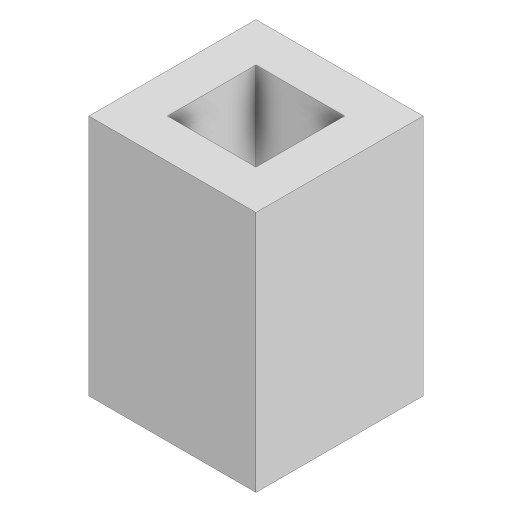
# Autodesk Inventor part: Tampa_fotometro
Saved by Autodesk Inventor 2024.3 (Build 283343000, 343)
## iProperties
Created: 2024-05-16
Part Number: Tampa_fotometro
Material: Genérico
Document SubType Name: Modeling
Designer: barof
Density: 1 g/cm^3
Appearance: Padrão
Author: barof
## iProperties of the stored document Tampa_fotometro_3DPrint.ipt
Created: 2025-02-10
Part Number: Tampa_fotometro_3DPrint
Material: Genérico
Document SubType Name: Modeling
Designer: barof
Density: 1 g/cm^3
Appearance: Padrão
Author: barof
Autodesk Inventor part; units mm, degrees
ref_plane "YZ Plane" through (0, 0, 0) normal (1, 0, 0) x (0, 1, 0)
ref_plane "XZ Plane" through (0, 0, 0) normal (0, 1, 0) x (-1, 0, 0)
ref_plane "XY Plane" through (0, 0, 0) normal (0, 0, 1) x (1, 0, 0)
sketch "Esboço1" plane through (0, 0, 0) normal (0, 1, 0) x (-1, 0, 0)
  line L0 (0, 0) -> (-25.5, 0)
  line L1 (-25.5, 0) -> (-25.5, -25.5)
  line L2 (-25.5, -25.5) -> (0, -25.5)
  line L3 (0, -25.5) -> (0, 0)
  line L4 (-6, -19.5) -> (-19.5, -19.5)
  line L5 (-19.5, -19.5) -> (-19.5, -6)
  line L6 (-19.5, -6) -> (-6, -6)
  line L7 (-6, -6) -> (-6, -19.5)
  point P0 (-25.5, -12.75)
  point P1 (-19.5, -12.75)
  point P2 (-12.75, 0)
  point P3 (-12.75, -6)
  point P4 (-6, -12.75)
  dimension "d0" = 6
  dimension "d1" = 6
  dimension "d2" = 6
  dimension "d3" = 6
  dimension "d4" = 13.5
  dimension "d5" = 13.5
  constraints: 16 end point, 5 midpoint, 4 parallel, 2 horizontal, 2 perpendicular
  measures "d0" distance of point (-25.5, -12.75) point (-19.5, -12.75)
  measures "d1" distance of point (-12.75, 0) point (-12.75, -6)
  measures "d2" distance from line of point (-6, -12.75) L3
  measures "d3" distance between parallel lines of L2 L4
  measures "d4" distance of L4.end L5.end
  measures "d5" distance of L5.end L6.end
extrude "Extrusão1" add sketch "Esboço1" along normal blind 3 contours L4 L5 L6 L7
extrude "Extrusão2" add sketch "Esboço1" along normal blind 37
